Autodesk Fusion 360 part; units mm, degrees
note: some values were not read from the file. Set by a fixed rule: which sketch regions a step uses.
(part 2 of 2)
sketch "Skizze4" plane through (0, 0, 1.75) normal (0, 0, 1) x (-1, 0, 0)
  line L0 (-2, -130.5) -> (-2, -72.5)
  line L1 (-2, -72.5) -> (-91.5, -72.5)
  line L2 (-91.5, -72.5) -> (-91.5, -130.5)
  line L3 (-91.5, -130.5) -> (-2, -130.5)
  spline S0 degree 3 poles (-43.772559, -124.775188) (-42.095616, -125.151202) (-40.510469, -124.950672) (-38.977301, -124.756798) knots 0 0 0 0 1 1 1 1
  spline S1 degree 3 poles (-38.977301, -124.756798) (-37.668121, -124.591157) (-36.43177, -124.434933) (-35.283741, -124.671227) knots 0 0 0 0 1 1 1 1
  spline S2 degree 3 poles (-35.283741, -124.671227) (-32.562292, -125.231413) (-29.575156, -123.494386) (-27.27678, -121.918359) knots 0 0 0 0 1 1 1 1
  spline S3 degree 3 poles (-27.27678, -121.918359) (-24.712862, -120.160189) (-24.349153, -118.257668) (-24.115174, -115.761653) knots 0 0 0 0 1 1 1 1
  spline S4 degree 3 poles (-24.115174, -115.761653) (-24.102577, -115.626709) (-24.096062, -115.488871) (-24.096062, -115.352044) knots 0 0 0 0 1 1 1 1
  spline S5 degree 3 poles (-24.096062, -115.352044) (-24.096062, -113.67713) (-25.033424, -112.278037) (-25.536999, -111.526292) knots 0 0 0 0 1 1 1 1
  spline S6 degree 3 poles (-25.536999, -111.526292) (-25.667599, -111.331264) (-25.802687, -111.129714) (-25.814559, -111.070641) knots 0 0 0 0 1 1 1 1
  spline S7 degree 3 poles (-25.814559, -111.070641) (-25.833237, -110.977108) (-25.836133, -110.758189) (-25.839897, -110.481204) knots 0 0 0 0 1 1 1 1
  spline S8 degree 3 poles (-25.839897, -110.481204) (-25.849743, -109.73728) (-25.866393, -108.492388) (-26.183915, -107.01004) knots 0 0 0 0 1 1 1 1
  spline S9 degree 3 poles (-26.183915, -107.01004) (-26.493473, -105.565628) (-27.229145, -104.408187) (-27.823936, -104.429761) knots 0 0 0 0 1 1 1 1
  spline S10 degree 3 poles (-27.823936, -104.429761) (-28.049227, -104.437869) (-28.339529, -104.602638) (-28.442763, -105.34164) knots 0 0 0 0 1 1 1 1
  spline S11 degree 3 poles (-28.442763, -105.34164) (-28.659222, -106.890011) (-29.078675, -108.258988) (-29.415599, -109.358948) knots 0 0 0 0 1 1 1 1
  spline S12 degree 3 poles (-29.415599, -109.358948) (-29.482202, -109.576421) (-29.54475, -109.780428) (-29.600494, -109.969667) knots 0 0 0 0 1 1 1 1
  spline S13 degree 3 poles (-29.600494, -109.969667) (-29.951752, -111.159831) (-30.431726, -112.25921) (-32.421847, -112.635661) knots 0 0 0 0 1 1 1 1
  spline S14 degree 3 poles (-32.421847, -112.635661) (-33.805737, -112.897582) (-35.393636, -110.518126) (-36.794755, -108.418979) knots 0 0 0 0 1 1 1 1
  spline S15 degree 3 poles (-36.794755, -108.418979) (-37.375792, -107.548221) (-37.924686, -106.725966) (-38.462865, -106.063556) knots 0 0 0 0 1 1 1 1
  spline S16 degree 3 poles (-38.462865, -106.063556) (-40.339761, -103.753598) (-44.14365, -99.349123) (-45.480339, -97.938158) knots 0 0 0 0 1 1 1 1
  spline S17 degree 3 poles (-45.480339, -97.938158) (-46.747386, -96.600745) (-54.459121, -85.353413) (-55.93394, -82.330079) knots 0 0 0 0 1 1 1 1
  spline S18 degree 3 poles (-55.93394, -82.330079) (-57.441045, -79.240578) (-59.803565, -76.229552) (-61.312406, -75.475058) knots 0 0 0 0 1 1 1 1
  spline S19 degree 3 poles (-61.312406, -75.475058) (-61.650632, -75.305945) (-61.864921, -75.269747) (-62.006957, -75.357489) knots 0 0 0 0 1 1 1 1
  spline S20 degree 3 poles (-62.006957, -75.357489) (-62.068928, -75.395858) (-62.142767, -75.475058) (-62.142767, -75.63476) knots 0 0 0 0 1 1 1 1
  spline S21 degree 3 poles (-62.142767, -75.63476) (-62.142767, -75.824867) (-62.033164, -76.085197) (-61.926888, -76.309765) knots 0 0 0 0 1 1 1 1
  spline S22 degree 3 poles (-61.926888, -76.309765) (-61.954106, -76.310054) (-61.982054, -76.315122) (-62.010576, -76.326995) knots 0 0 0 0 1 1 1 1
  spline S23 degree 3 poles (-62.010576, -76.326995) (-62.172593, -76.394032) (-62.193298, -76.610056) (-62.193298, -76.790753) knots 0 0 0 0 1 1 1 1
  spline S24 degree 3 poles (-62.193298, -76.790753) (-62.193298, -77.284627) (-61.990449, -78.314075) (-61.647301, -79.569538) knots 0 0 0 0 1 1 1 1
  spline S25 degree 3 poles (-61.647301, -79.569538) (-61.980605, -79.118666) (-62.554404, -78.224016) (-63.07651, -77.410014) knots 0 0 0 0 1 1 1 1
  spline S26 degree 3 poles (-63.07651, -77.410014) (-65.141199, -74.192239) (-66.143863, -72.76332) (-66.628761, -72.80386) knots 0 0 0 0 1 1 1 1
  spline S27 degree 3 poles (-66.628761, -72.80386) (-66.897345, -72.826158) (-67.217473, -73.003669) (-67.217473, -73.722545) knots 0 0 0 0 1 1 1 1
  spline S28 degree 3 poles (-67.217473, -73.722545) (-67.217473, -74.163861) (-67.104105, -74.701606) (-67.013033, -75.1338) knots 0 0 0 0 1 1 1 1
  spline S29 degree 3 poles (-67.013033, -75.1338) (-66.965834, -75.358078) (-66.924855, -75.552385) (-66.909218, -75.686604) knots 0 0 0 0 1 1 1 1
  spline S30 degree 3 poles (-66.909218, -75.686604) (-67.011875, -75.637665) (-67.188372, -75.512133) (-67.313759, -75.423088) knots 0 0 0 0 1 1 1 1
  spline S31 degree 3 poles (-67.313759, -75.423088) (-67.719457, -75.134669) (-68.139056, -74.836404) (-68.404596, -75.04881) knots 0 0 0 0 1 1 1 1
  spline S32 degree 3 poles (-68.404596, -75.04881) (-68.484374, -75.112516) (-68.523178, -75.220963) (-68.523178, -75.379941) knots 0 0 0 0 1 1 1 1
  spline S33 degree 3 poles (-68.523178, -75.379941) (-68.523178, -75.855572) (-68.170326, -76.87141) (-67.82906, -77.853801) knots 0 0 0 0 1 1 1 1
  spline S34 degree 3 poles (-67.82906, -77.853801) (-67.585379, -78.555158) (-67.355311, -79.217566) (-67.275242, -79.617907) knots 0 0 0 0 1 1 1 1
  spline S35 degree 3 poles (-67.275242, -79.617907) (-67.153041, -80.229205) (-65.618425, -83.19245) (-64.134341, -86.057963) knots 0 0 0 0 1 1 1 1
  spline S36 degree 3 poles (-64.134341, -86.057963) (-63.027141, -88.195913) (-61.772259, -90.619097) (-61.743591, -90.879862) knots 0 0 0 0 1 1 1 1
  spline S37 degree 3 poles (-61.743591, -90.879862) (-61.743591, -91.387635) (-61.444315, -95.489935) (-60.704875, -98.077454) knots 0 0 0 0 1 1 1 1
  spline S38 degree 3 poles (-60.704875, -98.077454) (-60.540106, -98.654148) (-60.456563, -99.270225) (-60.456563, -99.908597) knots 0 0 0 0 1 1 1 1
  spline S39 degree 3 poles (-60.456563, -99.908597) (-60.456563, -101.460587) (-60.939145, -102.958716) (-61.418395, -104.242268) knots 0 0 0 0 1 1 1 1
  spline S40 degree 3 poles (-61.418395, -104.242268) (-61.730848, -104.234306) (-62.113671, -104.226487) (-62.583655, -104.218379) knots 0 0 0 0 1 1 1 1
  spline S41 degree 3 poles (-62.583655, -104.218379) (-63.872999, -104.196516) (-65.208384, -104.186815) (-65.561235, -104.190001) knots 0 0 0 0 1 1 1 1
  spline S42 degree 3 poles (-65.561235, -104.190001) (-66.054095, -104.194201) (-66.923844, -105.124901) (-68.098657, -106.439148) knots 0 0 0 0 1 1 1 1
  spline S43 degree 3 poles (-68.098657, -106.439148) (-68.581963, -106.979788) (-69.175306, -107.643356) (-69.388725, -107.765267) knots 0 0 0 0 1 1 1 1
  spline S44 degree 3 poles (-69.388725, -107.765267) (-69.525697, -107.545044) (-69.529749, -107.207397) (-69.534817, -106.788668) knots 0 0 0 0 1 1 1 1
  spline S45 degree 3 poles (-69.534817, -106.788668) (-69.54365, -106.057195) (-69.555668, -105.055547) (-70.34795, -104.016544) knots 0 0 0 0 1 1 1 1
  spline S46 degree 3 poles (-70.34795, -104.016544) (-70.809393, -103.411472) (-71.469192, -103.011421) (-71.790482, -102.920638) knots 0 0 0 0 1 1 1 1
  spline S47 degree 3 poles (-71.790482, -102.920638) (-71.820161, -102.912095) (-71.910367, -102.886759) (-71.984352, -102.942645) knots 0 0 0 0 1 1 1 1
  spline S48 degree 3 poles (-71.984352, -102.942645) (-72.025326, -102.973774) (-72.04893, -103.021555) (-72.04893, -103.073825) knots 0 0 0 0 1 1 1 1
  spline S49 degree 3 poles (-72.04893, -103.073825) (-72.04893, -103.117405) (-72.032714, -103.161278) (-71.999411, -103.208477) knots 0 0 0 0 1 1 1 1
  line L4 (-71.999411, -103.208477) -> (-71.923106, -103.315186)
  spline S50 degree 3 poles (-71.923106, -103.315186) (-71.680295, -103.654137) (-71.111564, -104.447724) (-70.949401, -104.873982) knots 0 0 0 0 1 1 1 1
  spline S51 degree 3 poles (-70.949401, -104.873982) (-70.73019, -105.450097) (-70.640854, -105.873313) (-70.640854, -106.335189) knots 0 0 0 0 1 1 1 1
  spline S52 degree 3 poles (-70.640854, -106.335189) (-70.640854, -106.941565) (-70.796646, -107.658269) (-71.084341, -108.768508) knots 0 0 0 0 1 1 1 1
  spline S53 degree 3 poles (-71.084341, -108.768508) (-71.260404, -109.448436) (-71.346121, -110.028894) (-71.346121, -110.543038) knots 0 0 0 0 1 1 1 1
  spline S54 degree 3 poles (-71.346121, -110.543038) (-71.346121, -111.211816) (-71.204518, -111.697437) (-71.054661, -112.21144) knots 0 0 0 0 1 1 1 1
  spline S55 degree 3 poles (-71.054661, -112.21144) (-70.880334, -112.809564) (-70.700073, -113.42781) (-70.700073, -114.438724) knots 0 0 0 0 1 1 1 1
  spline S56 degree 3 poles (-70.700073, -114.438724) (-70.700073, -114.626515) (-70.706444, -114.824587) (-70.719183, -115.027578) knots 0 0 0 0 1 1 1 1
  spline S57 degree 3 poles (-70.719183, -115.027578) (-70.788537, -116.135065) (-71.365231, -117.127306) (-71.642357, -117.604236) knots 0 0 0 0 1 1 1 1
  spline S58 degree 3 poles (-71.642357, -117.604236) (-71.761663, -117.809546) (-71.797715, -117.871659) (-71.797715, -117.938844) knots 0 0 0 0 1 1 1 1
  line L5 (-71.797715, -117.938844) -> (-71.793659, -118.041063)
  line L6 (-71.793659, -118.041063) -> (-71.708234, -118.079435)
  spline S59 degree 3 poles (-71.708234, -118.079435) (-71.596602, -118.129674) (-71.525657, -118.06655) (-71.184245, -117.763505) knots 0 0 0 0 1 1 1 1
  spline S60 degree 3 poles (-71.184245, -117.763505) (-70.611025, -117.254429) (-70.260347, -116.778073) (-70.033611, -116.317646) knots 0 0 0 0 1 1 1 1
  spline S61 degree 3 poles (-70.033611, -116.317646) (-69.978882, -116.599115) (-69.90388, -116.859013) (-69.825985, -117.126148) knots 0 0 0 0 1 1 1 1
  spline S62 degree 3 poles (-69.825985, -117.126148) (-69.651658, -117.724272) (-69.471397, -118.342518) (-69.471397, -119.353286) knots 0 0 0 0 1 1 1 1
  spline S63 degree 3 poles (-69.471397, -119.353286) (-69.471397, -119.541077) (-69.477768, -119.739149) (-69.490507, -119.94214) knots 0 0 0 0 1 1 1 1
  spline S64 degree 3 poles (-69.490507, -119.94214) (-69.559861, -121.049627) (-70.136555, -122.042009) (-70.413535, -122.518798) knots 0 0 0 0 1 1 1 1
  spline S65 degree 3 poles (-70.413535, -122.518798) (-70.532988, -122.724254) (-70.568893, -122.786367) (-70.568893, -122.853552) knots 0 0 0 0 1 1 1 1
  line L7 (-70.568893, -122.853552) -> (-70.564837, -122.955771)
  line L8 (-70.564837, -122.955771) -> (-70.479412, -122.994143)
  spline S66 degree 3 poles (-70.479412, -122.994143) (-70.367781, -123.044382) (-70.296835, -122.981258) (-69.955423, -122.678213) knots 0 0 0 0 1 1 1 1
  spline S67 degree 3 poles (-69.955423, -122.678213) (-68.74166, -121.600405) (-68.518106, -120.667241) (-68.380846, -119.727131) knots 0 0 0 0 1 1 1 1
  spline S68 degree 3 poles (-68.380846, -119.727131) (-68.327129, -119.357921) (-68.203046, -119.078767) (-68.079396, -119.048363) knots 0 0 0 0 1 1 1 1
  spline S69 degree 3 poles (-68.079396, -119.048363) (-67.978188, -119.023314) (-67.806905, -119.160428) (-67.621284, -119.415257) knots 0 0 0 0 1 1 1 1
  spline S70 degree 3 poles (-67.621284, -119.415257) (-67.292037, -119.867289) (-67.125093, -120.321923) (-67.125093, -120.766571) knots 0 0 0 0 1 1 1 1
  spline S71 degree 3 poles (-67.125093, -120.766571) (-67.125093, -121.554368) (-67.642277, -122.044475) (-67.8389, -122.097759) knots 0 0 0 0 1 1 1 1
  spline S72 degree 3 poles (-67.8389, -122.097759) (-67.92809, -122.121791) (-67.959656, -122.192308) (-67.959656, -122.245587) knots 0 0 0 0 1 1 1 1
  spline S73 degree 3 poles (-67.959656, -122.245587) (-67.959656, -122.299883) (-67.926645, -122.371553) (-67.833978, -122.39472) knots 0 0 0 0 1 1 1 1
  spline S74 degree 3 poles (-67.833978, -122.39472) (-67.660809, -122.4383) (-66.901972, -122.386033) (-66.558677, -121.745053) knots 0 0 0 0 1 1 1 1
  spline S75 degree 3 poles (-66.558677, -121.745053) (-66.387103, -121.424925) (-66.2927, -120.929459) (-66.2927, -120.349871) knots 0 0 0 0 1 1 1 1
  spline S76 degree 3 poles (-66.2927, -120.349871) (-66.2927, -118.98075) (-66.774265, -117.491164) (-67.597389, -116.263787) knots 0 0 0 0 1 1 1 1
  spline S77 degree 3 poles (-67.597389, -116.263787) (-67.547869, -116.01924) (-67.52123, -115.739361) (-67.52123, -115.435304) knots 0 0 0 0 1 1 1 1
  spline S78 degree 3 poles (-67.52123, -115.435304) (-67.52123, -115.350891) (-67.523837, -115.265899) (-67.527455, -115.180766) knots 0 0 0 0 1 1 1 1
  spline S79 degree 3 poles (-67.527455, -115.180766) (-66.689419, -114.132352) (-64.738823, -112.287453) (-64.075401, -112.181177) knots 0 0 0 0 1 1 1 1
  spline S80 degree 3 poles (-64.075401, -112.181177) (-63.637995, -112.111244) (-62.255985, -112.070412) (-60.919442, -112.070412) knots 0 0 0 0 1 1 1 1
  spline S81 degree 3 poles (-60.919442, -112.070412) (-60.914374, -112.070412) (-60.909598, -112.070412) (-60.90453, -112.070412) knots 0 0 0 0 1 1 1 1
  spline S82 degree 3 poles (-60.90453, -112.070412) (-60.472479, -112.939144) (-59.963403, -113.821052) (-59.36166, -114.843839) knots 0 0 0 0 1 1 1 1
  spline S83 degree 3 poles (-59.36166, -114.843839) (-56.350642, -119.96357) (-46.868431, -124.081216) (-43.772559, -124.775188) knots 0 0 0 0 1 1 1 1
  spline S84 degree 3 poles (-62.359517, -109.118316) (-63.275741, -109.106878) (-64.071646, -109.102245) (-64.332697, -109.104561) knots 0 0 0 0 1 1 1 1
  spline S85 degree 3 poles (-64.332697, -109.104561) (-64.825415, -109.108904) (-65.695159, -110.039459) (-66.869972, -111.353564) knots 0 0 0 0 1 1 1 1
  spline S86 degree 3 poles (-66.869972, -111.353564) (-67.32678, -111.864668) (-67.881319, -112.484797) (-68.12109, -112.654347) knots 0 0 0 0 1 1 1 1
  spline S87 degree 3 poles (-68.12109, -112.654347) (-68.17003, -112.539384) (-68.221428, -112.425291) (-68.275869, -112.312356) knots 0 0 0 0 1 1 1 1
  spline S88 degree 3 poles (-68.275869, -112.312356) (-68.300194, -112.137451) (-68.303379, -111.933157) (-68.306132, -111.703376) knots 0 0 0 0 1 1 1 1
  spline S89 degree 3 poles (-68.306132, -111.703376) (-68.311925, -111.229773) (-68.32032, -110.642797) (-68.539531, -110.005873) knots 0 0 0 0 1 1 1 1
  spline S90 degree 3 poles (-68.539531, -110.005873) (-67.619976, -108.941386) (-65.915669, -107.382882) (-65.304519, -107.284859) knots 0 0 0 0 1 1 1 1
  spline S91 degree 3 poles (-65.304519, -107.284859) (-64.973098, -107.231867) (-64.098864, -107.212465) (-63.113141, -107.20146) knots 0 0 0 0 1 1 1 1
  spline S92 degree 3 poles (-63.113141, -107.20146) (-62.968211, -107.624241) (-62.737272, -108.253927) (-62.359517, -109.118316) knots 0 0 0 0 1 1 1 1
extrude "Extrusion5" [suppressed]
extrude "Extrusion8" [suppressed]
equation "d28 = 88 mm + 1.5 mm"
equation "d32 = 88 mm + 1.5 mm"
